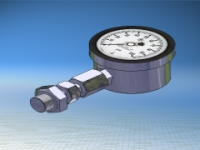
# Autodesk Inventor part: Pressure Gauge - 0.75 in BSP
Saved by Autodesk Inventor 2020 (Build 240152000, 152)
## iProperties
Created: 2009-08-11
Part Number: Pressure Gauge - 0.75 in BSP
Cost Center: 0.5 kg
Material: Generic
Description: Pressure Gauge-PN16 BSPT Thread
Document SubType Name: Modeling
Standard: NA
Designer: Demir Ali
Standards Organization: CUSTOM
Language: en-US
Size Designation: 19.05
Categories: <MemberInstance><Categories><Category DisplayName="Tube &amp; Pipe" InternalName="4347fa0f-2144-441d-94cd-e3e15c92b736" Mnemonic="TUBEANDPIPE"><CategoryParameter DisplayName="InLineGroups" InternalName="d60be647-bc43-4c18-a13f-9fe4115f8e64" Mnemonic="INLINEGROUPS"/><CategoryParameter DisplayName="Number of Connections" InternalName="04e9c83a-9e20-4a98-a7e1-e8abe87a2846" Mnemonic="NUM_CONNECTIONS"/><CategoryParameter DisplayName="NameOfComponent" InternalName="9c74ad13-48a1-45fe-b0f7-5447561f444a" Mnemonic="NAMEOFCOMPONENT"/><CategoryParameter DisplayName="SKey" InternalName="3da84699-049a-4bc2-a65a-6696b77c242f" Mnemonic="SKEY"/><CategoryParameter DisplayName="ITEM-CODE" InternalName="99cc3b15-24d9-4d38-aac7-792cfbc57acf" Mnemonic="ITEMCODE"/><CategoryParameter DisplayName="ISOGEN Description" InternalName="7aa3ba45-b821-4467-8584-f9e6f15f2a7d" Mnemonic="ISOGENDESC"/><Category DisplayName="Fittings" InternalName="ed6b26c4-72b8-4f31-9b63-f85ae8f932e4" Mnemonic="FITTINGS"><CategoryParameter DisplayName="Connections" InternalName="dbd721e8-e885-4eea-9011-b5acfd9f61de" Mnemonic="FIT_CONNECTIONS"><CategoryParameter DisplayName="NominalSize" InternalName="3f94edc7-e459-48db-8f02-8eebf8cffccd" Mnemonic="NS"/><CategoryParameter DisplayName="FlipDirection" InternalName="d55dedc0-f14a-4283-86b4-a4eeb253c8aa" Mnemonic="FLIPDIRECTION"/><CategoryParameter DisplayName="DisplayName" InternalName="50f521dd-e050-43f7-9895-6b30ea7ed42e" Mnemonic="DISPLAYNAME"/><CategoryParameter DisplayName="Female" InternalName="b366bcb5-a500-4bad-84bb-22f956216d69" Mnemonic="FEMALE"/><CategoryParameter DisplayName="EndTreatment" InternalName="d7f11516-3374-45ca-b1c7-4b2d63244ae2" Mnemonic="ENDTREATMENT"/><CategoryParameter DisplayName="Fixed" InternalName="9142902a-6a8a-446d-9eb8-4b7ce7d245ef" Mnemonic="FIXED"/><CategoryParameter DisplayName="MaxEngagement" InternalName="34fdf028-8797-436e-ba07-ca3dee15bd9b" Mnemonic="MAXENGAGEMENT"/><CategoryParameter DisplayName="MinEngagement [% of MaxEngagement]" InternalName="7ec1bde5-73f0-45b1-98d8-365a6c67f8ad" Mnemonic="MINENGAGEMENT"/><CategoryParameter DisplayName="ScheduleNumber" InternalName="d6161c62-eb59-4495-a086-874847c10866" Mnemonic="SN"/><CategoryParameter DisplayName="Max Mating Pipe Size" InternalName="e73ef66b-c04b-45ac-9b32-f712653e25ee" Mnemonic="MXMPS"/><CategoryParameter DisplayName="Min Mating Pipe Size" InternalName="11f51b32-3e37-4310-abf7-f1318a1fd129" Mnemonic="MNMPS"/><CategoryParameter DisplayName="Cut Mating Pipe" InternalName="53a63a6e-53d8-4ca9-8880-037731d1cceb" Mnemonic="CMP"/><CategoryParameter DisplayName="Gender Neutral" InternalName="628bd5f1-acad-44e2-9d91-af996ab74fc2" Mnemonic="NEUTRAL"/></CategoryParameter><Category DisplayName="Plugs" InternalName="9e68204e-4216-46be-a59d-a9118e32c8ef" Mnemonic="Plug"/></Category></Category><Category DisplayName="DataType" InternalName="23b78d0f-2648-40c6-8793-ca6db495c9e8" Mnemonic="DATATYPE"><CategoryParameter DisplayName="DisplayName" InternalName="05415f3d-3907-474b-a020-eb9d644f4cf3" Mnemonic="DISPLAYNAME"/><CategoryParameter DisplayName="InternalName" InternalName="cf1d0246-76d9-4b4a-8305-fa0409afb5c1" Mnemonic="INTERNALNAME"/><CategoryParameter DisplayName="Folder Name" InternalName="3f06958e-8713-4116-9be7-ed6184ecc97b" Mnemonic="FOLDERNAME"/><CategoryParameter DisplayName="Family Version" InternalName="914462f6-6e19-4b14-ba84-155b9680b1d0" Mnemonic="FAMILYREVISION"/><CategoryParameter DisplayName="ClipFormat" InternalName="bc51e27b-3422-4e78-93ef-cec197ddf230" Mnemonic="CLIPFORMAT"/><CategoryParameter DisplayName="IsMetric" InternalName="e2385c5b-1ea4-4823-96a8-8de651266ec3" Mnemonic="ISMETRIC"/><CategoryParameter DisplayName="Description" InternalName="13903e3d-64b1-4950-80da-f627842ea37f" Mnemonic="DESCRIPTION"/><CategoryParameter DisplayName="StdsOrg" InternalName="8f5914e1-4693-403f-8ab5-d37768198c9d" Mnemonic="STDSORG"/><CategoryParameter DisplayName="Standard" InternalName="0c0a119c-1e12-4c84-803f-101930972f5e" Mnemonic="STANDARD"/><CategoryParameter DisplayName="Manufacturer" InternalName="cd6c7a72-a28a-4e50-99a9-2c7f4e13e5ad" Mnemonic="MANUFACTURER"/><CategoryParameter DisplayName="Member Revision" InternalName="a65d44b9-392f-4f4f-857b-e4b3d54996fe" Mnemonic="MEMBERREVISION"/><CategoryParameter DisplayName="Standard Revision" InternalName="91d5a463-65c2-4fde-b823-3b7fea5e8e17" Mnemonic="STANDARDREVISION"/><CategoryParameter DisplayName="Revision Guid" InternalName="45a75005-10b1-4dfc-8d6d-dfe629f0b93c" Mnemonic="REVISIONGUID"/><CategoryParameter DisplayName="Designation" InternalName="2675968c-4ce5-49e0-a4f5-552d29089031" Mnemonic="DESIGNATION"/><CategoryParameter DisplayName="FileName" InternalName="8b46a4cc-9585-4fed-90c3-899f57e09a73" Mnemonic="FILENAME"/><CategoryParameter DisplayName="Default Row" InternalName="2af9ec52-faaa-4026-b378-f9fa4afca842" Mnemonic="DEFAULTROW"/><Category DisplayName="Part" InternalName="c0e0b642-3bcb-4cc8-9e80-f96d35c4afa4" Mnemonic="PART"><CategoryParameter DisplayName="Material" InternalName="818a152a-d3c3-49ca-80ee-df7d91421b8e" Mnemonic="MATERIAL"/><CategoryParameter DisplayName="Material Key" InternalName="5c9a8adb-dd2b-4535-b97f-0a94a95fe41f" Mnemonic="MATERIALKEY"/><CategoryParameter DisplayName="Part Number" InternalName="016b6077-bfbe-49bd-92c9-d8d59c39c941" Mnemonic="PARTNUMBER"/><CategoryParameter DisplayName="Stock Number" InternalName="4dba7c1c-e26c-444e-836c-b08b433409a8" Mnemonic="STOCKNUMBER"/></Category></Category></Categories><FamilyTemplate Id="Pressure Gauge-PN16 BSPT Thread"><FamilyTemplateParameters><FamilyTemplateParameter ObjectType="kModelParameterObject" ValueType="xs:double" Id="1" ObjectReferenceKey="Connection_dia"/><FamilyTemplateParameter ObjectType="kUserParameterObject" ValueType="xs:double" Id="2" ObjectReferenceKey="d38"/><FamilyTemplateParameter ObjectType="kUserParameterObject" ValueType="xs:double" Id="3" ObjectReferenceKey="d43"/><FamilyTemplateParameter ObjectType="kUserParameterObject" ValueType="xs:double" Id="4" ObjectReferenceKey="d45"/><FamilyTemplateParameter ObjectType="kUserParameterObject" ValueType="xs:double" Id="5" ObjectReferenceKey="d47"/><FamilyTemplateParameter ObjectType="kUserParameterObject" ValueType="xs:double" Id="6" ObjectReferenceKey="d65"/><FamilyTemplateParameter ObjectType="kUserParameterObject" ValueType="xs:double" Id="7" ObjectReferenceKey="d66"/><FamilyTemplateParameter ObjectType="kUserParameterObject" ValueType="xs:double" Id="8" ObjectReferenceKey="d67"/><FamilyTemplateParameter ObjectType="kThreadFeatureObject" ValueType="xs:string" Id="10" ObjectReferenceKey="10020000100000008a080000000000008000000000000000" SubObjectId="ThreadInfo"><FamilyTemplateParameter ObjectType="" ValueType="xs:string" Id="11" SubObjectId="NominalDiameter"/></FamilyTemplateParameter><FamilyTemplateParameter ObjectType="kPartComponentDefinitionObject" ValueType="xs:string" Id="13" SubObjectId="Material"/><FamilyTemplateParameter ObjectType="kPropertyObject" ValueType="xs:string" Id="37" ObjectReferenceKey="{32853F0F-3444-11d1-9E93-0060B03C1CA6}" SubObjectId="5"/><FamilyTemplateParameter ObjectType="kPropertyObject" ValueType="xs:string" Id="38" ObjectReferenceKey="{32853F0F-3444-11d1-9E93-0060B03C1CA6}" SubObjectId="52"/></FamilyTemplateParameters></FamilyTemplate><CategoryParameterMap><ParamToTemplateMap><ParamToTemplate CategoryParameter="//CategoryParameter[@InternalName='cf1d0246-76d9-4b4a-8305-fa0409afb5c1']" ConstantValue="42c53df4-0369-4463-bd16-c8aadd4f66b9"/><ParamToTemplate CategoryParameter="//CategoryParameter[@InternalName='45a75005-10b1-4dfc-8d6d-dfe629f0b93c']" ConstantValue="8651ea61-2d8d-489e-8ce3-06bd9ac0c395"/><ParamToTemplate CategoryParameter="//CategoryParameter[@InternalName='3f06958e-8713-4116-9be7-ed6184ecc97b']" ConstantValue="Pressure Gauge-PN16 BSPT Thread"/><ParamToTemplate CategoryParameter="//CategoryParameter[@InternalName='8f5914e1-4693-403f-8ab5-d37768198c9d']" ConstantValue="CUSTOM"/><ParamToTemplate CategoryParameter="//CategoryParameter[@InternalName='0c0a119c-1e12-4c84-803f-101930972f5e']" ConstantValue="NA"/><ParamToTemplate CategoryParameter="//CategoryParameter[@InternalName='91d5a463-65c2-4fde-b823-3b7fea5e8e17']" TemplateParameter="20"/><ParamToTemplate CategoryParameter="//CategoryParameter[@InternalName='cd6c7a72-a28a-4e50-99a9-2c7f4e13e5ad']" TemplateParameter="21"/><ParamToTemplate CategoryParameter="//CategoryParameter[@InternalName='13903e3d-64b1-4950-80da-f627842ea37f']" ConstantValue="Pressure Gauge-PN16 BSPT Thread"/><ParamToTemplate CategoryParameter="//CategoryParameter[@InternalName='05415f3d-3907-474b-a020-eb9d644f4cf3']" ConstantValue="Pressure Gauge-PN16 BSPT Thread"/><ParamToTemplate CategoryParameter="//CategoryParameter[@InternalName='914462f6-6e19-4b14-ba84-155b9680b1d0']" ConstantValue="11"/><ParamToTemplate CategoryParameter="//CategoryParameter[@InternalName='bc51e27b-3422-4e78-93ef-cec197ddf230']" ConstantValue="CF_INVENTOR.STDPARTS"/><ParamToTemplate CategoryParameter="//CategoryParameter[@InternalName='e2385c5b-1ea4-4823-96a8-8de651266ec3']" ConstantValue="true"/><ParamToTemplate CategoryParameter="//CategoryParameter[@InternalName='2af9ec52-faaa-4026-b378-f9fa4afca842']" ConstantValue="1"/><ParamToTemplate CategoryParameter="//CategoryParameter[@InternalName='d60be647-bc43-4c18-a13f-9fe4115f8e64']" ConstantValue="0"/><ParamToTemplate CategoryParameter="//CategoryParameter[@InternalName='04e9c83a-9e20-4a98-a7e1-e8abe87a2846']" ConstantValue="1"/><ParamToTemplate CategoryParameter="//CategoryParameter[@InternalName='dbd721e8-e885-4eea-9011-b5acfd9f61de'][1]/CategoryParameter[@InternalName='d55dedc0-f14a-4283-86b4-a4eeb253c8aa']" ConstantValue="false"/><ParamToTemplate CategoryParameter="//CategoryParameter[@InternalName='dbd721e8-e885-4eea-9011-b5acfd9f61de'][1]/CategoryParameter[@InternalName='50f521dd-e050-43f7-9895-6b30ea7ed42e']" ConstantValue="Connection1"/><ParamToTemplate CategoryParameter="//CategoryParameter[@InternalName='dbd721e8-e885-4eea-9011-b5acfd9f61de'][1]/CategoryParameter[@InternalName='628bd5f1-acad-44e2-9d91-af996ab74fc2']" ConstantValue="true"/><ParamToTemplate CategoryParameter="//CategoryParameter[@InternalName='dbd721e8-e885-4eea-9011-b5acfd9f61de'][1]/CategoryParameter[@InternalName='b366bcb5-a500-4bad-84bb-22f956216d69']" ConstantValue="false"/><ParamToTemplate CategoryParameter="//CategoryParameter[@InternalName='dbd721e8-e885-4eea-9011-b5acfd9f61de'][1]/CategoryParameter[@InternalName='d7f11516-3374-45ca-b1c7-4b2d63244ae2']" ConstantValue="Threaded"/><ParamToTemplate CategoryParameter="//CategoryParameter[@InternalName='dbd721e8-e885-4eea-9011-b5acfd9f61de'][1]/CategoryParameter[@InternalName='9142902a-6a8a-446d-9eb8-4b7ce7d245ef']" ConstantValue="false"/><ParamToTemplate CategoryParameter="//CategoryParameter[@InternalName='dbd721e8-e885-4eea-9011-b5acfd9f61de'][1]/CategoryParameter[@InternalName='34fdf028-8797-436e-ba07-ca3dee15bd9b']" ConstantValue="0.500000"/><ParamToTemplate CategoryParameter="//CategoryParameter[@InternalName='dbd721e8-e885-4eea-9011-b5acfd9f61de'][1]/CategoryParameter[@InternalName='7ec1bde5-73f0-45b1-98d8-365a6c67f8ad']" ConstantValue="50.000000"/><ParamToTemplate CategoryParameter="//CategoryParameter[@InternalName='8b46a4cc-9585-4fed-90c3-899f57e09a73']" ConstantValue="Pressure Gauge - 0.75 in BSP"/><ParamToTemplate CategoryParameter="//CategoryParameter[@InternalName='a65d44b9-392f-4f4f-857b-e4b3d54996fe']" ConstantValue="ca5525d7-f5dd-4413-8055-8c6a595e1576"/><ParamToTemplate CategoryParameter="//CategoryParameter[@InternalName='a65d44b9-392f-4f4f-857b-e4b3d54996fe']" ConstantValue="ca5525d7-f5dd-4413-8055-8c6a595e1576"/><ParamToTemplate CategoryParameter="//CategoryParameter[@InternalName='dbd721e8-e885-4eea-9011-b5acfd9f61de'][1]/CategoryParameter[@InternalName='3f94edc7-e459-48db-8f02-8eebf8cffccd']" TemplateParameter="1"/><ParamToTemplate CategoryParameter="//CategoryParameter[@InternalName='2675968c-4ce5-49e0-a4f5-552d29089031']" TemplateParameter="38"/><ParamToTemplate CategoryParameter="//CategoryParameter[@InternalName='818a152a-d3c3-49ca-80ee-df7d91421b8e']" TemplateParameter="13"/><ParamToTemplate CategoryParameter="//CategoryParameter[@InternalName='016b6077-bfbe-49bd-92c9-d8d59c39c941']" TemplateParameter="37"/></ParamToTemplateMap></CategoryParameterMap></MemberInstance>
Mass: 495.129 g
Surface Area: 484.46 cm^2
Volume: 495.129 cm^3
Density: 1 g/cm^3
Appearance: Chrome - Polished Blue
TotalMass: 0.5 kg
IsCustomPart: 0
Author: Demir Ali
Autodesk Inventor part; units mm, degrees
sketch "Sketch1" plane through (0, 0, 0) normal (0, 0, 1) x (1, 0, 0)
  circle A0 centre (0, 0) radius 50
  dimension "d0" = 100
  constraints: 1 centre point, 1 coincident
  measures "d0" diameter of A0
extrude "Extrusion1" add sketch "Sketch1" along normal blind 15
decal "Decal1"
sketch "Sketch3" plane through (0, 0, 0) normal (0, 0, -1) x (-1, 0, 0)
  circle A0 centre (0, 0) radius 50 projected
  circle A1 centre (0, 0) radius 45
  dimension "d17" = 90
  constraints: 1 centre point, 1 coincident, 1 concentric
  measures "d17" diameter of A1
extrude "Extrusion2" add sketch "Sketch3" along normal blind 48 contours A1
fillet "Fillet1" radius 2 1 edges at (45, 0, -48)
ref_plane "Work Plane1" through (0, -45, 0) normal (0, 1, 0) x (-1, 0, 0)
sketch "Sketch4" plane through (0, -45, 0) normal (0, 1, 0) x (-1, 0, 0)
  line L0 (-13.1053, -16.2891) -> (-1.3144, -7.9639)
  line L1 (-1.3144, -7.9639) -> (11.7909, -14.0125)
  line L2 (11.7909, -14.0125) -> (13.1053, -28.3863)
  line L3 (13.1053, -28.3863) -> (1.3144, -36.7115)
  line L4 (1.3144, -36.7115) -> (-11.7909, -30.6629)
  line L5 (-11.7909, -30.6629) -> (-13.1053, -16.2891)
  point P0 (0, -22.3377)
  point P1 (0, 0)
  dimension "d28" = 25
  constraints: 12 end point, 1 vertical alignment, 11 other
  measures "d28" distance between parallel lines of L3 L0
extrude "Extrusion3" add sketch "Sketch4" against normal blind 10
sketch "Sketch5" plane through (0, -55, 0) normal (0, -1, 0) x (1, 0, 0)
  line L0 (13.1053, -16.2891) -> (11.7909, -30.6629) projected
  line L1 (-1.3144, -36.7115) -> (-13.1053, -28.3863) projected
  circle A0 centre (0, -22.3377) radius 7.5
  dimension "d31" = 12.5
  dimension "d32" = 12.5
  dimension "d33" = 15
  constraints: 1 centre point
  measures "d31" distance from line of A0.centre L0
  measures "d32" distance from line of A0.centre L1
  measures "d33" diameter of A0
extrude "Extrusion4" add sketch "Sketch5" along normal blind 60
sketch "Sketch6" plane through (0, -115, -22.3377) normal (0, -1, 0) x (1, 0, 0)
  circle A0 centre (0, 0) radius 7.5 projected
  line L0 (-8.6603, 15) -> (8.6603, 15)
  line L1 (8.6603, 15) -> (17.3205, 0)
  line L2 (17.3205, 0) -> (8.6603, -15)
  line L3 (8.6603, -15) -> (-8.6603, -15)
  line L4 (-8.6603, -15) -> (-17.3205, 0)
  line L5 (-17.3205, 0) -> (-8.6603, 15)
  dimension "d38" = 30
  constraints: 12 end point, 1 coincident, 1 horizontal, 13 other
  measures "d38" distance between parallel lines of L3 L0
extrude "Extrusion5" add sketch "Sketch6" against normal blind 60 contours A0 | L0 L1 L2 L3 L4 L5
ref_plane "Work Plane2" through (0, -100, 0) normal (0, -1, 0) x (1, 0, 0)
sketch "Sketch7" plane through (0, -100, 0) normal (0, -1, 0) x (1, 0, 0)
  line L0 (-8.6603, -7.3377) -> (8.6603, -7.3377) projected
  line L1 (-17.3205, -22.3377) -> (-8.6603, -7.3377) projected
  line L2 (-8.6603, -37.3377) -> (-17.3205, -22.3377) projected
  line L3 (8.6603, -37.3377) -> (-8.6603, -37.3377) projected
  line L4 (17.3205, -22.3377) -> (8.6603, -37.3377) projected
  line L5 (8.6603, -7.3377) -> (17.3205, -22.3377) projected
extrude "Extrusion6" cut sketch "Sketch7" against normal blind 10
extrude "Extrusion7" add sketch "Sketch5" along normal blind 70
sketch "Sketch9" plane through (0, -125, -22.3377) normal (0, -1, 0) x (1, 0, 0)
  circle A0 centre (0, 0) radius 7.5 projected
  circle A1 centre (0, 0) radius 9.525
  dimension "Connection_dia" = 19.05
  constraints: 1 centre point, 1 coincident
  measures "Connection_dia" diameter of A1
extrude "Extrusion9" add sketch "Sketch9" along normal blind 30 contours A0 | A1
sketch "Sketch8" plane through (0, -125, -22.3377) normal (0, -1, 0) x (1, 0, 0)
  circle A0 centre (0, 0) radius 7.5 projected
  line L0 (-20, 11.547) -> (0, 23.094)
  line L1 (0, 23.094) -> (20, 11.547)
  line L2 (20, 11.547) -> (20, -11.547)
  line L3 (20, -11.547) -> (0, -23.094)
  line L4 (0, -23.094) -> (-20, -11.547)
  line L5 (-20, -11.547) -> (-20, 11.547)
  dimension "d47" = 40
  constraints: 12 end point, 1 coincident, 1 vertical, 13 other
  measures "d47" distance between parallel lines of L2 L5
extrude "Extrusion8" add sketch "Sketch8" along normal blind 15 contours A0 | L0 L1 L2 L3 L4 L5
thread "Thread1" size "R 3/4" standard "BSP Taper" full length
chamfer "Chamfer1" distance 0.5 angle 45 1 edges at (-9.525, -155, -22.3377)
ref_plane "Work Plane3" through (0, -55, -22.3377) normal (0, 0, 1) x (0, -1, 0)
sketch "Sketch11" plane through (0, -55, -22.3377) normal (0, 0, 1) x (0, -1, 0)
  line L0 (35, 17.3205) -> (0, 17.3205) projected
  line L1 (60, 17.3205) -> (45, 17.3205) projected
  line L2 (70, 20) -> (85, 20) projected
  line L3 (0, 17.3205) -> (0, 15.6324)
  line L4 (0, 15.6324) -> (2.0608, 17.3205)
  line L5 (35, 17.3205) -> (35, 14.8266)
  line L6 (35, 14.8266) -> (34.0634, 17.3205)
  line L7 (45, 17.3205) -> (45, 15.6324)
  line L8 (45, 15.6324) -> (47.0608, 17.3205)
  line L9 (60, 17.3205) -> (60, 15.2597)
  line L10 (60, 15.2597) -> (58.3119, 17.3205)
  line L11 (70, 24.731) -> (70, 17.183)
  line L12 (70, 17.183) -> (72.664, 24.731)
  line L13 (72.664, 24.731) -> (70, 24.731)
  line L14 (85, 24.731) -> (85, 17.183)
  line L15 (85, 17.183) -> (82.336, 24.731)
  line L16 (82.336, 24.731) -> (85, 24.731)
  line L17 (85, 0) -> (85, 20) projected
  line L18 (70, 0) -> (70, 20) projected
  line L19 (-143, 0) -> (123, 0) projected
  dimension "d65" = 24.731
  dimension "d66" = 2.817
  dimension "d67" = 2.664
  constraints: 28 end point, 6 equal length, 6 parallel, 4 perpendicular, 4 point on line, 3 collinear
  measures "d65" distance between parallel lines of L16 L19
  measures "d66" distance from line of L2 L14.end
  measures "d67" distance from line of L17 L15.end
revolve "Revolution1" cut sketch "Sketch11" angle 360 about axis through (0, -55, -22.3377) along (0, -1, 0) contours L5 L6 L0 | L4 L3 L0 | L9 L10 L1 | L8 L7 L1 | L11 L13 L12 L2 | L2 L12 L11 | L15 L16 L14 L2 | L2 L14 L15
sketch "Sketch2" plane through (0, 0, 15) normal (0, 0, 1) x (1, 0, 0)
  line L0 (-54.0441, 52.7497) -> (50.9716, 52.7497) construction
  line L1 (50.9716, 52.7497) -> (50.9716, -52.266) construction
  line L2 (50.9716, -52.266) -> (-54.0441, -52.266) construction
  line L3 (-54.0441, -52.266) -> (-54.0441, 52.7497) construction
  constraints: 2 other
body "Solid1"
